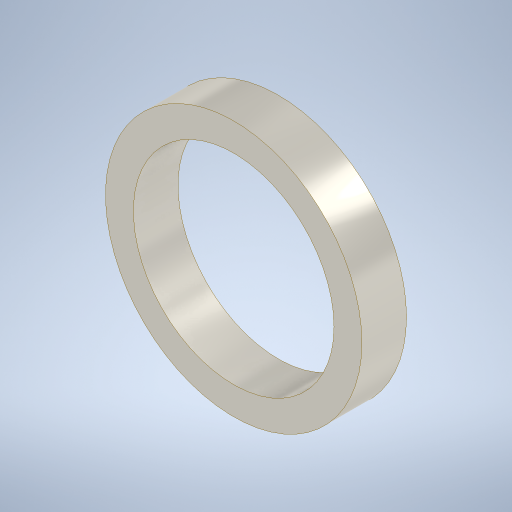
# Autodesk Inventor part: kolo_z
Saved by Autodesk Inventor 2023 (Build 270158000, 158)
## iProperties
Created: 2023-03-28
Part Number: kolo_z
Material: Tytan
Document SubType Name: Modeling
Designer: krzys
Density: 4.51 g/cm^3
Appearance: Tytan
Author: krzys
Autodesk Inventor part; units mm, degrees
ref_plane "YZ Plane" through (0, 0, 0) normal (1, 0, 0) x (0, 1, 0)
ref_plane "XZ Plane" through (0, 0, 0) normal (0, 1, 0) x (-1, 0, 0)
ref_plane "XY Plane" through (0, 0, 0) normal (0, 0, 1) x (1, 0, 0)
sketch "Szkic1" plane through (0, 0, 0) normal (0, 0, 1) x (1, 0, 0)
  circle A0 centre (0, 0) radius 50
  circle A1 centre (0, 0) radius 45
  circle A2 centre (0, 0) radius 57.5
  dimension "d0" = 100
  dimension "d1" = 90
  dimension "d2" = 115
  constraints: 3 centre point, 3 coincident
  measures "d0" diameter of A0
  measures "d1" diameter of A1
  measures "d2" diameter of A2
extrude "Wyciągnięcie proste1" add sketch "Szkic1" along normal blind 20 contours A0 | A2
